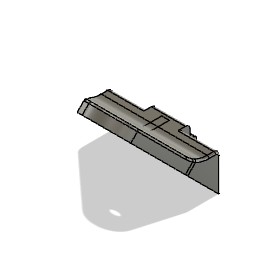
webcam-mount (Autodesk Fusion 360 design; units mm, degrees)
Autodesk Fusion 360 part; units mm, degrees
note: some values were not read from the file. Chosen so that the rebuilt part matches the saved one: which pieces of a blend or face edit are solid. Set by a fixed rule: which sketch regions a step uses.
sketch "2020-front-mount" plane through (0, 0, 0) normal (0, 0, 1) x (1, 0, 0)
  line L0 (-29, 10) -> (29, 10)
  line L1 (29, 10) -> (29, -10)
  line L2 (29, -10) -> (-29, -10)
  line L3 (-29, -10) -> (-29, 10)
  circle A0 centre (-20, 0) radius 2.75
  circle A1 centre (20, 0) radius 2.75
  line L4 (0, 10) -> (0, -10) construction
  line L5 (-9, 10) -> (9, 10)
  line L6 (9, 10) -> (9, -10)
  line L7 (9, -10) -> (-9, -10)
  line L8 (-9, -10) -> (-9, 10)
  line L9 (-9, 3) -> (9, 3)
  line L10 (9, 3) -> (9, -3)
  line L11 (9, -3) -> (-9, -3)
  line L12 (-9, -3) -> (-9, 3)
  line L13 (-29, 0) -> (29, 0) construction
  dimension "d5" = 5.5
  dimension "d6" = 40
  dimension "d7" = 18
  dimension "d8" = 58
  dimension "d9" = 20
  dimension "d10" = 6
  constraint horizontal L0
  constraint vertical L1
  constraint horizontal L2
  constraint vertical L3
  constraint equal A0 A1
  constraint collinear origin A0.centre A1.centre
  constraint midpoint L0 L4.start
  constraint midpoint L2 L4.end
  constraint coincident origin L4
  constraint symmetric A0.centre A1.centre L4
  constraint horizontal L5
  constraint vertical L6
  constraint horizontal L7
  constraint vertical L8
  constraint coincident L2 L6.end
  constraint coincident L0 L5.start
  constraint horizontal L9
  constraint vertical L10
  constraint horizontal L11
  constraint vertical L12
  constraint coincident L6 L10.end
  constraint midpoint L3 L13.start
  constraint midpoint L1 L13.end
  constraint coincident origin L13
  constraint coincident L8 L9.start
  constraint symmetric L9 L11 L13
  constraint symmetric L4 L6 L8
  measures "d5" diameter of A0
  measures "d6" distance of A0.centre A1.centre
  measures "d7" distance of L5.start L5.end
  measures "d8" distance of L0.start L0.end
  measures "d9" distance of L0.start L2.end
  measures "d10" distance of L9.start L11.end
extrude "Extrude1" add sketch "2020-front-mount" along normal blind 4 makes body 1
extrude "Extrude3" add sketch "2020-front-mount" against normal blind 8 draft -5 contours L6 L8 L9 L10 L11 L12 bodies 1
extrude "Extrude2" add sketch "2020-front-mount" against normal blind 4 contours L0 L5 L6 L8 L9 | L6 L8 L9 L10 L11 L12 | L2 L6 L7 L8 L11 bodies 1
sketch "2020-base-mount" plane through (0, 0, 0) normal (0, 1, 0) x (1, 0, 0)
  line L0 (29, -4) -> (-29, -4)
  line L1 (0, 0) -> (0, 24) construction
  circle A0 centre (0, 14) radius 1.75
  line L2 (9, 0) -> (9, 24)
  line L3 (-9, 0) -> (-9, 24)
  line L4 (29, 0) -> (9, 0)
  line L5 (-29, 0) -> (-9, 0)
  line L6 (-9, 24) -> (9, 24)
  line L7 (29, -4) -> (29, 0)
  line L8 (-29, -4) -> (-29, 0)
  line L9 (27.5, 0) -> (9, 0) construction
  line L10 (-9, 0) -> (-29, 0) construction
  point P0 (29, -4)
  point P1 (-29, -4)
  point P2 (29, 0)
  dimension "d18" = 3.5
  dimension "d19" = 14
  dimension "d20" = 10
  dimension "d21" = 18
  constraint horizontal L0
  constraint coincident L0.start L7.start
  constraint coincident L0.end L8.start
  constraint coincident L1 A0.centre
  constraint coincident L3.start L9
  constraint coincident P2 L4.start
  constraint perpendicular L2 L4
  constraint perpendicular L3 L5
  constraint perpendicular L2 L6
  constraint perpendicular L4 L7
  constraint coincident P1 L0.end
  constraint perpendicular L5 L8
  constraint coincident L1.end L6
  constraint collinear L9 L10
  constraint horizontal L5
  constraint symmetric L1 L2 L3
  constraint coincident L1.start origin
  measures "d18" diameter of A0
  measures "d19" vertical distance of L9.start A0.centre
  measures "d20" distance of L1.end A0.centre
  measures "d21" distance of L2.end L3.end
sketch "Sketch19" plane through (0, 10, 0) normal (0, 1, 0) x (-1, 0, 0)
  line L0 (9, 0) -> (29, 0)
  line L1 (29, 0) -> (29, 4)
  line L2 (29, 4) -> (-29, 4)
  line L3 (-29, 4) -> (-29, 0)
  line L4 (-9, 0) -> (-9, -4)
  line L5 (-9, -4) -> (9, -4)
  line L6 (9, -4) -> (9, 0)
  line L7 (29, 0) -> (-29, 0)
  line L8 (-29, 0) -> (-29, 15)
  line L9 (-29, 15) -> (29, 15)
  line L10 (29, 15) -> (29, 0)
  line L11 (-29, 0) -> (-9, 0)
  dimension "d73" = 11
  constraint horizontal L7
  constraint vertical L8
  constraint horizontal L9
  constraint vertical L10
  constraint coincident L0.end L1.start
  constraint coincident L3.end L7.end
  measures "d73" distance of L1.end L9.end
extrude "Extrude18" add sketch "Sketch19" against normal blind 4 contours L2 L8 L9 L10 bodies 1
ref_plane "WorkPlane1" through (0, 10, 15) normal (0, -0.707107, 0.707107) x (-1, 0, 0)
sketch "mount-plate" plane through (0, 4.5, 9.5) normal (0, -0.707107, 0.707107) x (1, 0, 0)
  line L0 (-2.7232, 57.4516) -> (31.0842, 48.3929)
  line L1 (31.0842, 48.3929) -> (22.802, 17.4833)
  line L2 (22.802, 17.4833) -> (-11.0054, 26.542)
  line L3 (-11.0054, 26.542) -> (-2.7232, 57.4516)
  line L4 (-2.7232, 57.4516) -> (22.802, 17.4833) construction
  line L5 (31.0842, 48.3929) -> (-11.0054, 26.542) construction
  circle A0 centre (10.0394, 37.4674) radius 3.675
  line L6 (-8.9213, 67.1567) -> (41.3044, 53.6988)
  line L7 (41.3044, 53.6988) -> (29, 7.7782)
  line L8 (29, 7.7782) -> (-21.2256, 21.2361)
  line L9 (-21.2256, 21.2361) -> (-8.9213, 67.1567)
  line L10 (-8.9213, 67.1567) -> (-2.7232, 57.4516) construction
  line L11 (41.3044, 53.6988) -> (31.0842, 48.3929) construction
  line L12 (29, 7.7782) -> (22.802, 17.4833) construction
  line L13 (-21.2256, 21.2361) -> (-11.0054, 26.542) construction
  line L14 (0, 0) -> (14.1805, 52.9222) construction
  line L15 (0, 68.017) -> (0, 0) construction
  line L16 (-21.2256, 21.2361) -> (-29, 7.7782)
  line L17 (29, 7.7782) -> (-29, 7.7782)
  circle A1 centre (10.0394, 37.4674) radius 12.5
  line L18 (0.1868, 45.1601) -> (-29, 7.7782)
  line L19 (22.2761, 40.0194) -> (29, 7.7782)
  point P0 (-29, 0)
  point P1 (29, 0)
  point P2 (31.5014, 3.8613)
  point P3 (30.162, 2.2063)
  point P4 (29, 7.7782)
  point P5 (-29, 7.7782)
  dimension "d1" = 35
  dimension "d2" = 32
  dimension "d3" = 7.35
  dimension "d27" = 15
  dimension "d52" = 25
  constraint parallel L4 L10
  constraint parallel L5 L11
  constraint parallel L4 L12
  constraint coincident L4 A0.centre
  constraint coincident L5 A0.centre
  constraint coincident L14.start L15.end
  constraint perpendicular L8 L14
  constraint coincident A0.centre L14
  constraint coincident L8.end L9.start
  constraint perpendicular L8 L9
  constraint perpendicular L7 L8
  constraint perpendicular L6 L7
  constraint parallel L3 L9
  constraint parallel L0 L6
  constraint parallel L1 L7
  constraint parallel L2 L8
  constraint coincident L0 L14.end
  constraint vertical L15
  constraint concentric A0 A1
  constraint coincident A1 L18.start
  constraint tangent A1 L18
  constraint coincident A1 L19.start
  constraint tangent A1 L19
  constraint coincident L19 P3
  constraint coincident L12 P2
  constraint coincident P4 L7.end
  constraint coincident P5 L16.end
  measures "d1" distance of L0.start L0.end
  measures "d2" distance of L0.end L1.end
  measures "d3" diameter of A0
  measures "d27" angle of L14 L15
  measures "d52" diameter of A1
extrude "Extrude15" add sketch "mount-plate" against normal blind 2 separate body contours L1 L2 L3 A1 L18 L19 | L1 L2 L3 L8 L18 L19 | A1 | L8 L17 L18 makes body 2
extrude "Extrude20" add 1 faces at (6.4188, 19.1826, 24.1826) along direction (0, -0.707107, 0.707107) blind 4 on bodies 2 bodies 2 1
sketch "Sketch5" plane through (29, 0, 0) normal (1, 0, 0) x (0, 0, -1)
  line L0 (0, -10) -> (0, 10)
  line L1 (0, 10) -> (-15, 10)
  line L2 (-4, 6) -> (-4, -10)
  line L3 (-15, 10) -> (-12.1716, 10)
  line L4 (-12.1716, 10) -> (-13.5858, 11.4142)
  line L5 (-13.5858, 11.4142) -> (-15, 10)
  line L6 (-36.3838, 34.2122) -> (-13.5858, 11.4142)
  line L7 (-15, 10) -> (-15, 6)
  line L8 (-15, 6) -> (-17.8284, 7.1716)
  line L9 (-17.8284, 7.1716) -> (-15, 10)
  line L10 (-4, -10) -> (0, -10)
  point P0 (-13.5858, 11.4142)
  point P1 (-17.8284, 7.1716)
  point P2 (-15, 6)
  constraint coincident L1.end L3.start
  constraint perpendicular L0 L3
  constraint parallel L4 L6
  constraint coincident L3.end L4.start
  constraint perpendicular L3 L7
  constraint parallel L5 L9
  constraint coincident P1 L8.end
  constraint coincident P2 L7.end
extrude "Extrude6" add sketch "Sketch5" against normal blind 58 bodies 2
sketch "Sketch20" plane through (0, -5.3284, 5.3284) normal (0, -0.707107, 0.707107) x (1, 0, 0)
  circle A0 centre (9.9059, 46.8688) radius 3.675
  line L0 (0.0156, 54.5128) -> (-29, 16.9706)
  line L1 (29, 16.9706) -> (22.1358, 49.4532)
  arc A1 (22.1358, 49.4532) -> (0.0156, 54.5128) centre (9.9059, 46.8688) ccw
  line L2 (-50, 70) -> (58.9643, 70)
  line L3 (58.9643, 70) -> (58.9643, -47.879)
  line L4 (58.9643, -47.879) -> (-50, -47.879)
  line L5 (-50, -47.879) -> (-50, 70)
  line L6 (-29, 16.9706) -> (29, 16.9706)
  circle A2 centre (10.0394, 47.3669) radius 3.675
  line L7 (0.1868, 55.0596) -> (-29, 17.6777)
  line L8 (-29, 17.6777) -> (29, 17.6777)
  line L9 (29, 17.6777) -> (22.2761, 49.9189)
  arc A3 (22.2761, 49.9189) -> (0.1868, 55.0596) centre (10.0394, 47.3669) ccw
  constraint horizontal L2
  constraint vertical L3
  constraint horizontal L4
  constraint vertical L5
extrude "Extrude21" cut sketch "Sketch20" along normal blind 10 contours L2 L3 L4 L5 bodies 2
sketch "Sketch21" plane through (29, 0, 0) normal (1, 0, 0) x (0, 0, -1)
  line L0 (-4, -6.6569) -> (-0.6569, -10)
  line L1 (0, -10) -> (0, 10)
  line L2 (0, 10) -> (-12.1716, 10)
  line L3 (-12.1716, 10) -> (-13.5858, 11.4142)
  line L4 (-13.5858, 11.4142) -> (-17.8284, 7.1716)
  line L5 (-17.8284, 7.1716) -> (-15, 6)
  line L6 (-15, 6) -> (-4, 6)
  line L7 (-4, 6) -> (-4, -6.6569)
  line L8 (-17.8284, 7.1716) -> (-4, -6.6569)
  line L9 (-17.8284, 7.1716) -> (-4, 7.1716)
  line L10 (-4, 7.1716) -> (-4, -6.6569)
  line L11 (-12.1716, 10) -> (-15, 10)
  line L12 (-15, 10) -> (-17.8284, 7.1716)
  line L13 (-12.1716, 10) -> (-4, 10)
  line L14 (-4, 10) -> (-4, 7.1716)
  line L15 (-15, 10) -> (-20.6569, 10)
  line L16 (-20.6569, 10) -> (-17.8284, 7.1716)
  line L17 (-17.8284, 7.1716) -> (-40.6264, 29.9696)
  line L18 (-4, -6.6569) -> (-0.6569, -10)
  line L19 (-4, 10) -> (0, 10)
  line L20 (-0.6569, -10) -> (0, -10.1562)
  line L21 (0, 10) -> (-0.6569, -10)
  line L22 (-0.6569, -10) -> (0, -10)
  constraint coincident L4.end L5.start
  constraint coincident L0.start L7.end
  constraint perpendicular L1 L9
  constraint perpendicular L9 L10
  constraint coincident L2.end L3.start
  constraint coincident L4 L11.end
  constraint parallel L2 L11
  constraint coincident L2 L13.end
  constraint coincident L13.end L14.start
  constraint vertical L14
  constraint parallel L11 L15
  constraint coincident L15.end L17
  constraint coincident L0.end L18.end
  constraint coincident L1.end L2.start
  constraint coincident L1 L20.end
extrude "Extrude22" add sketch "Sketch21" against normal blind 2 contours L5 L6 L7 L8 L10 | L5 L6 L9 L10 bodies 2
extrude "Extrude23" add sketch "Sketch21" along normal blind 2 from surface at -58 contours L5 L6 L7 L8 L10 | L5 L6 L9 L10 bodies 2
extrude "Extrude24" add sketch "Sketch21" along normal mid plane 4 from surface at -29 separate body contours L0 L2 L7 L10 L14 L18 L19 L21 | L5 L6 L7 L8 L10 | L5 L6 L9 L10 | L4 L12 L15 L16 L17 | L2 L4 L9 L11 L12 L13 L14 makes body 3
fillet "Fillet16" radius 1 5 edges at (0, -6.6569, 4) (0, 6, 4) (0, -10, -4) (0, -2.3001, -8) (0, 2.3001, -8) on bodies 1 2
fillet "Fillet17" radius 10 2 edges at (0, 6, 15) (0, 7.1716, 17.8284) on bodies 2
fillet "Fillet18" radius 15 1 edges at (0, 10, 12.1716) on bodies 2
fillet "Fillet19" radius 7.5 2 edges at (29, 9.5064, 15.4936) (-29, 9.5064, 15.4936) on bodies 2
fillet "Fillet20" radius 2.5 3 edges at (0, 10, -4) (-19, 10, 0) (19, 10, 0) on bodies 2
chamfer "Chamfer1" distance 0.8 angle 45 2 edges at (6.6131, 29.1047, 39.7616) (6.6131, 31.468, 33.6396) on bodies 2
fillet "Fillet21" radius 1 15 edges at (-29, -1.25, 0) (-29, 9.2678, 0.7322) (-29, 10, 4.2292) (-29, 10.186, 8.3135) (-28.6173, 11.734, 12.9582) (-26.5633, 13.6492, 15.7645) (-12.7618, 26.1203, 28.2919) (12.8727, 41.0165, 43.188) (25.1987, 24.3028, 26.4744) (28.4841, 13.2349, 15.2633) (28.9617, 11.8319, 13.1414) (29, 10.3722, 9.2793) (29, 10, 4.2292) (29, 9.2678, 0.7322) (29, -1.25, 0) on bodies 2
equation "d3 = ( 25.4 * 0.25 ) * 1 mm + 1 mm"
equation "d19 = 10 mm + 4 mm"
